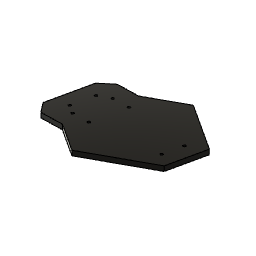
Board (Autodesk Fusion 360 design; units mm, degrees)
Autodesk Fusion 360 part; units mm, degrees
sketch "Esquisse3" plane through (0, 0, 0) normal (0, 1, 0) x (1, 0, 0)
  line L0 (-32.5, 271.1708) -> (-7.5, 296.1708)
  line L1 (-32.5, 261.1708) -> (127.5, 261.1708) construction
  line L2 (127.5, 216.1708) -> (-32.5, 216.1708) construction
  circle A0 centre (20, 261.1708) radius 3
  line L3 (-7.5, 296.1708) -> (102.5, 296.1708)
  circle A1 centre (89.5, 194.6708) radius 3
  line L4 (-32.5, 236.1708) -> (127.5, 236.1708) construction
  line L5 (0, -4.6657) -> (95, -4.6657)
  circle A2 centre (89.5, 236.1708) radius 3
  line L6 (47.5, 23.552) -> (47.5, 296.1708)
  circle A3 centre (5.5, 194.6708) radius 3
  line L7 (47.5, 30.3343) -> (47.5, -4.6657) construction
  line L8 (-44.913, 194.6708) -> (139.913, 194.6708) construction
  line L9 (-80, 133.8984) -> (0, -4.6657)
  line L10 (95, -4.6657) -> (175, 133.8984)
  line L11 (23.75, 67.2637) -> (23.75, -4.6657) construction
  line L12 (71.25, 67.8004) -> (71.25, 0) construction
  line L13 (-32.5, 216.1708) -> (-80, 133.8984)
  line L14 (127.5, 271.1708) -> (127.5, 216.1708)
  line L15 (102.5, 296.1708) -> (127.5, 271.1708)
  line L16 (-32.5, 216.1708) -> (-32.5, 271.1708)
  line L17 (-32.5, 271.1708) -> (127.5, 271.1708) construction
  line L18 (-20.2073, 30.3343) -> (115.2073, 30.3343) construction
  line L19 (175, 133.8984) -> (127.5, 216.1708)
  circle A4 centre (75, 261.1708) radius 3
  circle A5 centre (5.5, 236.1708) radius 3
  circle A6 centre (23.75, 30.3343) radius 3
  circle A7 centre (71.25, 30.3343) radius 3
  line L20 (5.5, 300.8365) -> (5.5, 171.5052) construction
  line L21 (89.5, 296.1708) -> (89.5, 171.5052) construction
  line L22 (20, 296.1708) -> (20, 171.5052) construction
  line L23 (75, 296.1708) -> (75, 171.5052) construction
  point P0 (0, -4.6657)
  dimension "d12" = 95
  dimension "d60" = 120
  dimension "d18" = 120
  dimension "d63" = 160
  dimension "d65" = 25
  dimension "d66" = 25
  dimension "d35" = 35
  dimension "d70" = 6
  dimension "d71" = 6
  dimension "d72" = 6
  dimension "d56" = 6
  dimension "d74" = 6
  dimension "d75" = 6
  dimension "d79" = 101.5
  dimension "d80" = 23.75
  dimension "d67" = 23.75
  dimension "d88" = 80
  dimension "d89" = 60
  dimension "d90" = 25
  dimension "d95" = 95
  dimension "d96" = 160
  dimension "d97" = 35
  dimension "d98" = 6
  dimension "d99" = 6
  dimension "d100" = 38
  dimension "d101" = 38
  dimension "d102" = 52.5
  dimension "d103" = 52.5
  constraint coincident P0 L5.start
  constraint horizontal L5
  constraint horizontal L2
  constraint perpendicular L2 L16
  constraint parallel L2 L3
  constraint perpendicular L2 L14
  constraint coincident L15.end L14
  constraint coincident L1.start L16
  constraint coincident L1.end L14
  constraint perpendicular L1 L14
  constraint coincident L4.start L16
  constraint coincident L4.end L14
  constraint perpendicular L4 L14
  constraint coincident L8.start L13
  constraint coincident L8.end L19
  constraint coincident A0.centre L1
  constraint coincident A4.centre L1
  constraint coincident A5.centre L4
  constraint coincident A2.centre L4
  constraint coincident A3.centre L8
  constraint coincident A1.centre L8
  constraint coincident L18.start L9
  constraint coincident L18.end L10
  constraint perpendicular L16 L17
  constraint midpoint L7.start L18
  constraint midpoint L7.end L5
  constraint coincident L11.end L5
  constraint perpendicular L5 L11
  constraint perpendicular L12 L18
  constraint coincident L6.start L7
  constraint perpendicular L6 L18
  constraint midpoint L6.end L3
  constraint coincident L11 A6.centre
  constraint coincident L18 A6.centre
  constraint coincident L18 A7.centre
  constraint coincident L12 A7.centre
  constraint coincident L3 L21.start
  constraint perpendicular L8 L21
  constraint coincident L3 L22.start
  constraint perpendicular L8 L22
  constraint coincident L3 L23.start
  constraint perpendicular L8 L23
  constraint midpoint A5.centre L20
  measures "d12" distance of P0 L5.end
  measures "d60" angle of L5 L10
  measures "d18" angle of L10 L19
  measures "d63" distance of L14 L16
  measures "d65" horizontal distance of L0.end L0.start
  measures "d66" horizontal distance of L14.start L3.end
  measures "d35" distance of L1 L3
  measures "d70" diameter of A0
  measures "d71" diameter of A4
  measures "d72" diameter of A5
  measures "d56" diameter of A2
  measures "d74" diameter of A3
  measures "d75" diameter of A1
  measures "d79" distance of L3 L8
  measures "d80" distance of L7 L11
  measures "d67" distance of L7 L12
  measures "d88" distance of L2 L3
  measures "d89" distance of L3 L4
  measures "d90" distance of L3 L17
  measures "d95" distance of L2.end L9.start
  measures "d96" distance of P0 L9.start
  measures "d97" distance of L5 L18
  measures "d98" diameter of A6
  measures "d99" diameter of A7
  measures "d100" distance of L16 L20
  measures "d101" distance of L14 L21
  measures "d102" distance of L16 L22
  measures "d103" distance of L14 L23
extrude "Extrusion5" add sketch "Esquisse3" along normal blind 10.12
equation "plaque0_l1_Ref = 160 mm"
equation "plaque0_l2_Ref = 95 mm"
equation "plaque_ep = 10.12 mm"
equation "support_prof = 80 mm"
equation "support_chanf = 25 mm"
equation "trou_butée_x = 38 mm"
equation "trou_butée_y = 60 mm"
equation "trou_diam = 6.05 mm"
equation "trou_butée_entraxe = 41.5 mm"
equation "trou_glissière_y = 35.025 mm"
equation "trou_glissière_entraxe = 55 mm"
equation "trou_glissière_x = 27.525 mm"
equation "d104 = plaque_ep"
